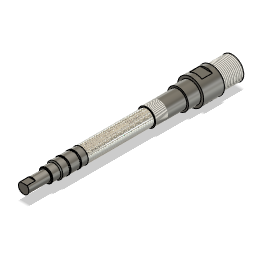
spindle_ER20 (Autodesk Fusion 360 design; units mm, degrees)
Autodesk Fusion 360 part; units mm, degrees
sketch "Sketch1" plane through (0, 0, 0) normal (0, 0, 1) x (1, 0, 0)
  circle A0 centre (0, 0) radius 12.5
  dimension "d1" = 25
  constraint coincident A0.centre origin
  measures "d1" diameter of A0
extrude "Extrude1" add sketch "Sketch1" along normal blind 20 makes body 1
sketch "Sketch2" plane through (0, 0, 20) normal (0, 0, 1) x (1, 0, 0)
  circle A0 centre (0, 0) radius 12.5
  circle A1 centre (0, 0) radius 10
  circle A2 centre (0, 0) radius 10
  circle A3 centre (0, 0) radius 8.5
  circle A4 centre (0, 0) radius 5
  circle A5 centre (0, 0) radius 8.5
  circle A6 centre (0, 0) radius 6.5
  circle A7 centre (0, 0) radius 8.5
  circle A8 centre (0, 0) radius 7.5
  circle A9 centre (0, 0) radius 8.5
  circle A10 centre (0, 0) radius 5
  circle A11 centre (0, 0) radius 12.5
  line L0 (-5.9372, -15) -> (5.9372, -15)
  line L1 (-5.9372, -15) -> (-5.9372, -5)
  line L2 (5.9372, -5) -> (-5.9372, -5)
  line L3 (5.9372, -5) -> (5.9372, -15)
  line L4 (-5.9372, -15) -> (5.9372, -15)
  line L5 (5.9372, -15) -> (5.9372, -5)
  line L6 (5.9372, -5) -> (-5.9372, -5)
  line L7 (-5.9372, -5) -> (-5.9372, -15)
  line L8 (-12.5, -20) -> (12.5, -20)
  line L9 (-12.5, 0) -> (12.5, 0)
  dimension "d4" = 20
  constraint concentric A0 A1
  measures "d4" diameter of A1
extrude "Extrude2" add sketch "Sketch2" along normal blind 12 contours A1 A2 A3 A5 A7 A9 L9 | A1 A2 A3 A5 A7 A9 L3 L5 L9 | A1 A2 A3 A5 A7 A9 L1 L7 L9 | A1 A2 A3 A5 A7 A9 L1 L3 L5 L7 | A3 A5 A7 A8 A9 L9 | A3 A5 A7 A8 A9 L2 L3 L5 L6 L9 | A3 A5 A7 A8 A9 L1 L2 L6 L7 L9 | A3 A5 A7 A8 A9 L1 L2 L3 L5 L6 L7 | A6 A8 L9 | A6 A8 L2 L6 L9 | A6 A8 L2 L6 L9 | A6 A8 L2 L6 | A4 A6 A10 L9 | A4 A6 A10 L2 L6 L9 | A4 A6 A10 L2 L6 L9 | A6 L2 L6 | A4 A10 L9 | A4 A10 L9 bodies 1
sketch "Sketch3" plane through (0, 0, 32) normal (0, 0, 1) x (1, 0, 0)
  circle A0 centre (0, 0) radius 10
  circle A1 centre (0, 0) radius 8.5
  dimension "d7" = 17
  constraint coincident A0.centre A1.centre
  measures "d7" diameter of A1
extrude "Extrude3" add sketch "Sketch3" along normal blind 30 contours A1 bodies 1
extrude "Extrude4" add 1 faces at (2.7075, 1.6235, 62) along direction (0, 0, 1) blind 118 separate body on bodies 1 makes body 2
sketch "Sketch4" plane through (0, 0, 180) normal (0, 0, 1) x (1, 0, 0)
  circle A0 centre (0, 0) radius 8.5
  circle A1 centre (0, 0) radius 5
  constraint concentric A0 A1
extrude "Extrude5" cut sketch "Sketch4" against normal blind 21 bodies 2
sketch "Sketch5" plane through (0, 0, 159) normal (0, 0, 1) x (1, 0, 0)
  circle A0 centre (0, 0) radius 5
  circle A1 centre (0, 0) radius 8.5
  circle A2 centre (0, 0) radius 6.5
  dimension "d14" = 13
  constraint concentric A0 A2
  measures "d14" diameter of A2
extrude "Extrude6" cut sketch "Sketch5" against normal blind 8 contours A1 bodies 2
sketch "Sketch6" plane through (0, 0, 151) normal (0, 0, 1) x (1, 0, 0)
  circle A0 centre (0, 0) radius 6.5
  circle A1 centre (0, 0) radius 8.5
  circle A2 centre (0, 0) radius 7.5
  dimension "d17" = 15
  constraint concentric A0 A2
  measures "d17" diameter of A2
extrude "Extrude7" cut sketch "Sketch6" against normal blind 8 contours A1 bodies 2
sketch "Sketch7" plane through (0, 0, 143) normal (0, 0, 1) x (1, 0, 0)
  circle A0 centre (0, 0) radius 7.5
  circle A1 centre (0, 0) radius 8.5
extrude "Extrude8" cut sketch "Sketch7" against normal blind 81 bodies 2
thread "Thread1" "ISO Metric profile 17.0 M17x1 6g" major diameter 16.884 minor diameter 15.7405 pitch 1 angle 60 resizes the face on face at (8.4578, -0.8463, 52) from (0, 0, 50) to (0, 0, 62) on bodies 1
sketch "Sketch8" plane through (0, 0, 180) normal (0, 0, 1) x (1, 0, 0)
  circle A0 centre (0, 0) radius 5
  line L0 (0, 0) -> (0, 3.8)
  line L1 (0, 3.8) -> (3.2496, 3.8)
  line L2 (0, 3.8) -> (-3.6202, 3.8)
  line L3 (-3.6202, 3.8) -> (-3.6202, 5.3015)
  line L4 (-3.6202, 5.3015) -> (0, 5.3015)
  line L5 (0, 5.3015) -> (0, 3.8)
  line L6 (0, 3.8) -> (3.4816, 3.8)
  line L7 (3.4816, 3.8) -> (3.4816, 5.3015)
  line L8 (3.4816, 5.3015) -> (0, 5.3015)
  line L9 (0, 5.3015) -> (0, 3.8)
  dimension "d24" = 3.8
  constraint coincident A0.centre L0.start
  constraint vertical L0
  constraint coincident A0 L1.end
  constraint perpendicular L0 L1
  constraint horizontal L2
  constraint vertical L3
  constraint horizontal L4
  constraint vertical L5
  constraint horizontal L6
  constraint vertical L7
  constraint horizontal L8
  constraint vertical L9
  measures "d24" distance of A0.centre L0.end
extrude "Extrude9" cut sketch "Sketch8" against normal blind 8 contours A0 L1 L5 L6 L9 | A0 L2 L5 L9 bodies 2
combine "Combine1" operation add target body 1 tool bodies 2
ref_plane "WorkPlane1" through (0, 0, 131.85) normal (0, 0, -1) x (-1, 0, 0)
sketch "Sketch9" plane through (0, 0, 131.85) normal (0, 0, -1) x (1, 0, 0)
  circle A0 centre (0, 0) radius 7.15
  circle A1 centre (0, 0) radius 7.5
  dimension "d28" = 14.3
  dimension "d29" = 15
  constraint coincident A0.centre A1.centre
  constraint concentric A0 A1
  measures "d28" diameter of A0
  measures "d29" diameter of A1
extrude "Extrude10" cut sketch "Sketch9" against normal blind 1.25 bodies 1
ref_plane "WorkPlane2" through (0, 0, 142.1) normal (0, 0, -1) x (1, 0, 0)
sketch "Sketch10" plane through (0, 0, 142.1) normal (0, 0, -1) x (1, 0, 0)
  circle A0 centre (0, 0) radius 7.15
  circle A1 centre (0, 0) radius 7.5
  dimension "d33" = 14.3
  dimension "d34" = 15
  constraint coincident A0.centre A1.centre
  constraint concentric A0 A1
  measures "d33" diameter of A0
  measures "d34" diameter of A1
extrude "Extrude11" cut sketch "Sketch10" against normal blind 1.25 bodies 1
chamfer "Chamfer1" distance 1 angle 45 1 edges at (-6.9925, -2.7121, 151) on bodies 1
chamfer "Chamfer2" distance 0.5 angle 45 1 edges at (-6.0601, -2.3505, 159) on bodies 1
extrude "Extrude12" add 1 faces at (1.9349, 2.0708, 0) along direction (0, 0, -1) blind 20 separate body on bodies 1 makes body 3
sketch "Sketch11" plane through (0, 0, -20) normal (0, 0, -1) x (-1, 0, 0)
  circle A0 centre (0, 0) radius 12.5
  circle A1 centre (0, 0) radius 8
  dimension "d41" = 16
  constraint coincident A0.centre A1.centre
  measures "d41" diameter of A1
ref_plane "WorkPlane3" through (0, 0, 0) normal (0, 0, -1) x (-1, 0, 0)
sketch "Sketch12" plane through (0, 0, 0) normal (0, 0, -1) x (1, 0, 0)
  circle A0 centre (0, 0) radius 6
  dimension "d43" = 12
  constraint coincident A0.centre origin
  measures "d43" diameter of A0
loft "Loft1" cut profiles "Sketch11", "Sketch12" section 1 contours A1 section 2 bodies 3
thread "Thread2" "ISO Metric profile 22.0 M22x1.5 6g" major diameter 21.85 minor diameter 20.137 pitch 1.5 angle 60 resizes the face on face at (12.4845, 0.6231, -13.3333) on bodies 3
ref_plane "WorkPlane4" through (0, 0, 10) normal (0, 0, -1) x (-1, 0, 0)
sketch "Sketch13" plane through (0, 0, 10) normal (0, 0, -1) x (1, 0, 0)
  line L0 (-10.925, -10) -> (10.925, -10)
  line L1 (10.925, -10) -> (10.925, 10)
  line L2 (10.925, 10) -> (-10.925, 10)
  line L3 (-10.925, 10) -> (-10.925, -10)
  line L4 (-10.925, -10) -> (10.925, 10) construction
  line L5 (10.925, -10) -> (-10.925, 10) construction
  circle A0 centre (0, 0) radius 12.5
  dimension "d45" = 21.85
  dimension "d46" = 25
  constraint perpendicular L0 L1
  constraint parallel L0 L2
  constraint parallel L1 L3
  constraint horizontal L0
  constraint coincident L4 A0.centre
  constraint coincident L5 A0.centre
  constraint coincident A0.centre origin
  measures "d45" distance of L1.end L2.end
  measures "d46" diameter of A0
extrude "Extrude13" cut sketch "Sketch13" along normal mid plane 10 contours L0 A0 | L2 A0 bodies 1
move_face "OffsetFaces1" offset 1 1 faces at (2.5, 10, 8.3333) on bodies 1
move_face "OffsetFaces2" offset 1 1 faces at (2.5, -10, 11.6667) on bodies 1
ref_plane "WorkPlane5" through (0, 0, 125.55) normal (0, 0, 1) x (-1, 0, 0)
sketch "Sketch14" plane through (0, 0, 125.55) normal (0, 0, 1) x (1, 0, 0)
  circle A0 centre (0, 0) radius 7.45
  circle A1 centre (0, 0) radius 7.5
  dimension "d52" = 14.9
  dimension "d53" = 15
  constraint coincident A0.centre A1.centre
  constraint concentric A0 A1
  measures "d52" diameter of A0
  measures "d53" diameter of A1
extrude "Extrude14" cut sketch "Sketch14" against normal blind 63.55 bodies 1
ref_plane "WorkPlane6" through (0, 0, 0) normal (0, 1, 0) x (0, 0, 1)
sketch "Sketch15" plane through (0, 0, 0) normal (0, 1, 0) x (1, 0, 0)
  line L0 (-5.9372, -15) -> (5.9372, -15)
  line L1 (-5.9372, -15) -> (-5.9372, -5)
  line L2 (5.9372, -5) -> (-5.9372, -5)
  line L3 (5.9372, -5) -> (5.9372, -15)
  line L4 (-5.9372, -15) -> (5.9372, -15)
  line L5 (5.9372, -15) -> (5.9372, -5)
  line L6 (5.9372, -5) -> (-5.9372, -5)
  line L7 (-5.9372, -5) -> (-5.9372, -15)
  line L8 (-12.5, -20) -> (12.5, -20)
  line L9 (-12.5, 0) -> (12.5, 0)
  line L10 (12.5, -20) -> (10, -20)
  line L11 (10, -20) -> (11, -20)
  line L12 (10, -20) -> (10, -21)
  line L13 (11, -20) -> (10.0887, -19.7558)
  line L14 (11, -20) -> (11.9434, -20) construction
  line L15 (10, -21) -> (9.4824, -19.0681)
  line L16 (10, -21) -> (12, -21) construction
  line L17 (10.0887, -19.7558) -> (9.634, -19.634)
  dimension "d57" = 165
  dimension "d58" = 105
  dimension "d59" = 2
  constraint coincident L8.end L10.start
  constraint coincident L8 L10.end
  constraint parallel L8 L10
  constraint coincident L10 L11.end
  constraint perpendicular L10 L12
  constraint horizontal L14
  constraint horizontal L16
  constraint coincident L15 L17.end
  constraint parallel L13 L17
  measures "d57" angle of L13 L14
  measures "d58" angle of L15 L16
  measures "d59" distance of L12.end L15.end
equation "d10 = 180 mm - 62 mm"
equation "d45 = 25 mm - 3.15 mm"
equation "d57 = 180 deg - 15 deg"
equation "d58 = 90 deg + 15 deg"
